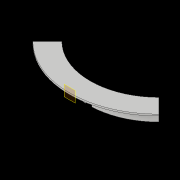
# Autodesk Inventor part: Layer2_Top_Quarter
Saved by Autodesk Inventor 2017 (Build 210142000, 142)
## iProperties
Created: 2017-01-16
Part Number: Layer2_Top_Quarter
Material: Generic
Document SubType Name: Modeling
Designer: David Kopala
Density: 1 g/cm^3
Appearance: Default
Author: David Kopala
Autodesk Inventor part; units mm, degrees
ref_plane "YZ Plane" through (0, 0, 0) normal (1, 0, 0) x (0, 1, 0)
ref_plane "XZ Plane" through (0, 0, 0) normal (0, 1, 0) x (-1, 0, 0)
ref_plane "XY Plane" through (0, 0, 0) normal (0, 0, 1) x (1, 0, 0)
sketch "Sketch1" plane through (0, 0, 0) normal (1, 0, 0) x (0, 1, 0)
  line L0 (0, 0) -> (50.8, 0)
  line L1 (0, 138.1125) -> (26.719, 138.1125)
  line L2 (0, 138.1125) -> (0, 169.8625)
  line L3 (0, 169.8625) -> (3.175, 169.8625)
  line L4 (3.175, 169.8625) -> (3.175, 141.2875)
  line L5 (22.9489, 141.2875) -> (60.325, 141.2875)
  line L6 (60.325, 141.2875) -> (60.325, 179.3875)
  line L7 (60.325, 179.3875) -> (63.5, 179.3875)
  line L8 (63.5, 179.3875) -> (63.5, 138.1125)
  line L9 (63.5, 138.1125) -> (35.6489, 138.1125)
  line L10 (29.2989, 139.7) -> (22.9489, 139.7)
  line L11 (22.9489, 139.7) -> (22.9489, 141.2875)
  line L12 (29.2989, 139.7) -> (35.6489, 139.7)
  line L13 (35.6489, 139.7) -> (35.6489, 138.1125)
  line L14 (29.2989, 164.2178) -> (29.2989, 141.2875)
  point P0 (62.1333, 179.3875)
  dimension "d0" = 50.8
  dimension "d1" = 138.1125
  dimension "d2" = 31.75
  dimension "d3" = 3.175
  dimension "d4" = 3.175
  dimension "d5" = 57.15
  dimension "d6" = 38.1
  dimension "d7" = 3.175
  dimension "d13" = 26.1239
  dimension "d14" = 1.5875
  dimension "d15" = 6.35
  dimension "d16" = 6.35
  constraints: 30 end point, 6 perpendicular, 4 horizontal, 3 point on line, 2 vertical, 1 collinear, 1 parallel
  measures "d0" distance of L0.start L0.end
  measures "d1" distance between parallel lines of L0 L1
  measures "d2" distance of L1.start L2.end
  measures "d3" distance of L2.end L3.end
  measures "d4" distance from line of L1 L4.end
  measures "d5" distance of L4.end L5.end
  measures "d6" distance of L5.end L6.end
  measures "d7" distance of L6.end L7.end
  measures "d13" distance from line of L14.start L4
  measures "d14" distance from line of L9 L10.start
  measures "d15" distance of L10.start L10.end
  measures "d16" distance of L10.start L12.end
revolve "Revolution1" add sketch "Sketch1" angle 360 about axis through (0, 0, 0) along (0, 1, 0)
ref_plane "Work Plane1" through (0, 62.1333, 179.3875) normal (0, 0, 1) x (1, 0, 0)
sketch "Sketch2" plane through (0, 62.1333, 179.3875) normal (0, 0, 1) x (1, 0, 0)
  arc A0 (6.35, -32.8344) -> (-6.35, -32.8344) centre (0, -32.8344) ccw
  line L0 (169.8625, -58.9583) -> (-169.8625, -58.9583) projected
  line L1 (-6.35, -32.8344) -> (-6.35, -39.1844)
  line L2 (141.2875, -39.1844) -> (-141.2875, -39.1844) projected
  line L3 (6.35, -32.8344) -> (6.35, -39.1844)
  line L4 (-6.35, -39.1844) -> (6.35, -39.1844)
  point P0 (0, -62.1333)
  dimension "d9" = 12.7
  dimension "d10" = 26.1239
  constraints: 6 end point, 2 point on circle, 2 point on line, 1 centre point, 1 parallel, 1 perpendicular, 1 vertical
  measures "d9" diameter of A0
  measures "d10" distance from line of A0.centre L0
extrude "Extrusion1" cut sketch "Sketch2" against normal through all
sketch "Sketch3" plane through (0, 63.5, 0) normal (0, 1, 0) x (1, 0, 0)
  line L0 (0, 0) -> (-271.4312, -271.4312)
  line L1 (0, 0) -> (383.8617, 0) construction
  line L2 (-271.4312, -271.4312) -> (-271.4312, 238.0261)
  line L3 (-271.4312, 238.0261) -> (250.2845, 238.0261)
  line L4 (0, 0) -> (271.4312, -271.4312)
  line L5 (0, 0) -> (383.8617, 0) construction
  line L6 (271.4312, -271.4312) -> (250.2845, 238.0261)
  dimension "d17" = 135
  dimension "d18" = 45
  constraints: 14 end point, 2 equal length, 2 horizontal, 1 perpendicular, 1 vertical
  measures "d17" angle of L0 L1
  measures "d18" angle of L4 L5
extrude "Extrusion2" cut sketch "Sketch3" against normal through all
body "Solid1"
